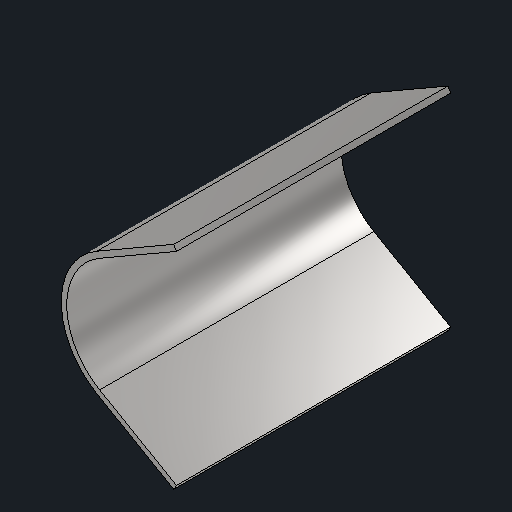
# Autodesk Inventor part: preanode-screen
Saved by Autodesk Inventor 2027.1 (Build 311270010, 270A)
## iProperties
Created: 2026-10-02
Part Number: preanode-screen
Material: Stainless Steel
Document SubType Name: Modeling
Designer: queezz
Density: 8 g/cm^3
Appearance: Semi-Polished
Author: queezz
Autodesk Inventor part; units mm, degrees
ref_plane "YZ Plane" through (0, 0, 0) normal (1, 0, 0) x (0, 1, 0)
ref_plane "XZ Plane" through (0, 0, 0) normal (0, 1, 0) x (-1, 0, 0)
ref_plane "XY Plane" through (0, 0, 0) normal (0, 0, 1) x (1, 0, 0)
sketch "Sketch1" plane through (0, 0, 0) normal (0, 0, 1) x (1, 0, 0)
  arc A0 (-3, 5.1962) -> (-3, -5.1962) centre (0, 0) ccw
  line L0 (-3, 5.1962) -> (4, 9.2376)
  line L1 (-3, -5.1962) -> (4, -9.2376)
  line L2 (0, 0) -> (4, 0)
  line L3 (3.75, 9.6706) -> (-3.25, 5.6292)
  arc A1 (-3.25, 5.6292) -> (-3.25, -5.6292) centre (0, 0) ccw
  line L4 (-3.25, -5.6292) -> (3.75, -9.6706)
  line L5 (3.75, 9.6706) -> (4, 9.2376)
  line L6 (4, -9.2376) -> (3.75, -9.6706)
  dimension "d0" = 12
  dimension "d1" = 4
  dimension "d2" = 60
  dimension "d3" = 0.5
  constraints: 14 end point, 4 point on circle, 3 vertical alignment, 2 centre point, 2 perpendicular, 2 tangent, 1 coincident, 1 horizontal, 2 other
  measures "d0" diameter of A0
  measures "d1" horizontal distance of L2.start L0.end
  measures "d2" angle of L1 L0
  measures "d3" distance between parallel lines of L0 L3
extrude "Extrusion1" add sketch "Sketch1" along normal blind 25
body "Solid1"
